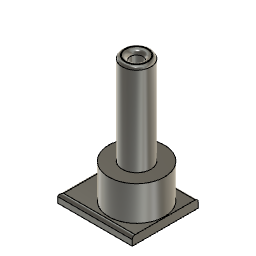
guide filament v5 (archive) (Autodesk Fusion 360 design; units mm, degrees)
Autodesk Fusion 360 part; units mm, degrees
note: some values were not read from the file. Chosen so that the rebuilt part matches the saved one: which face or edge a step refers to.
sketch "Esquisse1" plane through (0, 0, 0) normal (0, 0, 1) x (1, 0, 0)
  line L0 (0, 0) -> (16, 0)
  line L1 (16, 0) -> (16, 11.5)
  line L2 (16, 11.5) -> (0, 11.5)
  line L3 (0, 11.5) -> (0, 0)
  dimension "d1" = 16
  dimension "d2" = 11.5
  constraint horizontal L0
  constraint vertical L1
  constraint horizontal L2
  constraint vertical L3
  constraint coincident L0.start L3.end
  measures "d1" distance of L0.start L0.end
  measures "d2" distance of L0.start L2.end
extrude "Extrusion1" add sketch "Esquisse1" along normal blind 1.5
sketch "Esquisse2" plane through (0, 0, 1.5) normal (0, 0, 1) x (-1, 0, 0)
  line L0 (0, -11.5) -> (0, 0)
  line L1 (0, 0) -> (-16, 0)
  line L2 (-16, 0) -> (-16, -11.5)
  line L3 (-16, -11.5) -> (0, -11.5)
  line L4 (0, -5.75) -> (-8, -5.75)
  circle A0 centre (-8, -5.75) radius 4.85
  dimension "d5" = 9.7
  constraint midpoint L0 L4.start
  constraint perpendicular L0 L4
  constraint coincident L4.end A0.centre
  measures "d5" diameter of A0
extrude "Extrusion2" add sketch "Esquisse2" along normal blind 22 contours A0
sketch "Esquisse3" plane through (0, 0, 23.5) normal (0, 0, 1) x (-1, 0, 0)
  circle A0 centre (-8, -5.75) radius 4.85
  circle A1 centre (-8, -5.75) radius 2.5
  dimension "d8" = 5
  constraint concentric A0 A1
  measures "d8" diameter of A1
extrude "Extrusion3" cut sketch "Esquisse3" against normal blind 10
sketch "Esquisse4" plane through (0, 0, 23.5) normal (0, 0, 1) x (-1, 0, 0)
  circle A0 centre (-8, -5.75) radius 2.5
  circle A1 centre (-8, -5.75) radius 1.125
  dimension "d11" = 2.25
  constraint concentric A0 A1
  measures "d11" diameter of A1
extrude "Extrusion4" cut sketch "Esquisse4" against normal blind 33.5 contours A1
extrude "Extrusion5" cut 1 faces at (16, 3.8333, 0.5) along direction (-1, 0, 0) blind 3
fillet "Congé1" radius 0.75 1 edges at (9.0489, 5.3432, 23.5)
fillet "Congé2" radius 0.5 1 edges at (10.3308, 6.654, 23.5)
fillet "Congé3" radius 0.5 3 edges at (6.5, 11.5, 1.5) (6.5, 0, 1.5) (0, 5.75, 1.5)
extrude "Extrusion6" cut 1 faces at (3.9607, 6.1152, 13.5) along direction (0, 0, -1) blind 6
